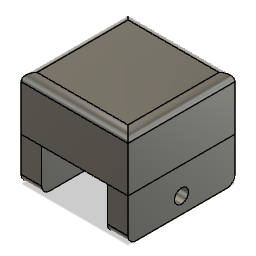
y-homing-stops v2 (Autodesk Fusion 360 design; units mm, degrees)
Autodesk Fusion 360 part; units mm, degrees
sketch "Sketch1" plane through (0, 0, 0) normal (0, 1, 0) x (1, 0, 0)
  line L0 (-10, 10) -> (10, 10)
  line L1 (10, 10) -> (10, -10)
  line L2 (10, -10) -> (-10, -10)
  line L3 (-10, -10) -> (-10, 10)
  line L4 (-10, 10) -> (10, -10) construction
  line L5 (10, 10) -> (-10, -10) construction
  line L6 (-6.125, 10) -> (6.125, 10)
  line L7 (6.125, 10) -> (6.125, -10)
  line L8 (6.125, -10) -> (-6.125, -10)
  line L9 (-6.125, -10) -> (-6.125, 10)
  line L10 (-6.125, 10) -> (6.125, -10) construction
  line L11 (6.125, 10) -> (-6.125, -10) construction
  dimension "d1" = 20
  dimension "d2" = 20
  dimension "d3" = 12.25
  constraint horizontal L0
  constraint vertical L1
  constraint horizontal L2
  constraint vertical L3
  constraint coincident origin L5
  constraint coincident origin L4
  constraint horizontal L6
  constraint vertical L7
  constraint horizontal L8
  constraint vertical L9
  constraint coincident L0 L6.start
  constraint coincident origin L11
  constraint coincident origin L10
  measures "d1" distance of L0.start L0.end
  measures "d2" distance of L0.start L2.end
  measures "d3" distance of L6.start L6.end
extrude "Extrude1" add sketch "Sketch1" along normal blind 8 contours L0 L2 L3 L9 | L0 L1 L2 L7 makes body 1 at (-10, 5.3333, 3.3333) makes body 2 at (10, 5.3333, -3.3333)
extrude "Extrude2" add sketch "Sketch1" along normal blind 10 from surface at 8 separate body makes body 3
sketch "Sketch2" plane through (10, 0, 0) normal (1, 0, 0) x (0, 0, -1)
  line L0 (-10, 0) -> (10, 0)
  line L1 (10, 0) -> (10, 8)
  line L2 (10, 8) -> (-10, 8)
  line L3 (-10, 8) -> (-10, 0)
  circle A0 centre (0, 3) radius 1.3
  dimension "d9" = 2.6
  dimension "d11" = 3
  constraint vertical A0.centre origin
  measures "d9" diameter of A0
  measures "d11" distance of origin A0.centre
extrude "Extrude3" cut sketch "Sketch2" along normal through all and the other way through all contours A0 bodies 1 2
fillet "Fillet1" radius 1.5 4 edges at (-8.0625, 0, 10) (-8.0625, 0, -10) (8.0625, 0, 10) (8.0625, 0, -10) on bodies 1 2
fillet "Fillet2" radius 1.5 4 edges at (0, 18, 10) (0, 18, -10) (-10, 18, 0) (10, 18, 0) on bodies 3
